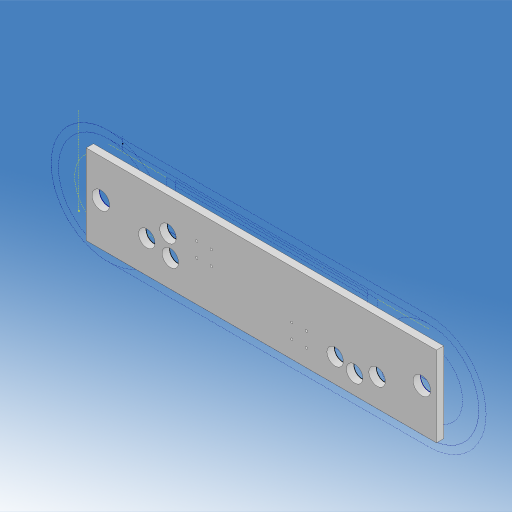
# Autodesk Inventor part: MasterSketch
Saved by Autodesk Inventor 2024 (Build 280153000, 153)
## iProperties
Created: 2024-03-21
Part Number: MasterSketch
Material: Generic
Document SubType Name: Modeling
Designer: seene
Density: 1 g/cm^3
Appearance: Default
Author: seene
Autodesk Inventor part; units mm, degrees
ref_plane "YZ Plane" through (0, 0, 0) normal (1, 0, 0) x (0, 1, 0)
ref_plane "XZ Plane" through (0, 0, 0) normal (0, 1, 0) x (-1, 0, 0)
ref_plane "XY Plane" through (0, 0, 0) normal (0, 0, 1) x (1, 0, 0)
sketch "Chassis" plane through (0, 0, 0) normal (0, 0, 1) x (1, 0, 0)
  line L0 (0, 0) -> (660.4, 0) construction
  line L1 (660.4, 0) -> (660.4, 152.4) construction
  line L2 (660.4, 152.4) -> (0, 152.4) construction
  line L3 (0, 152.4) -> (0, 0) construction
  line L4 (50.8, 127) -> (609.6, 127) construction
  line L5 (635, 101.6) -> (635, 50.8) construction
  line L6 (609.6, 25.4) -> (50.8, 25.4) construction
  line L7 (25.4, 50.8) -> (25.4, 101.6) construction
  arc A0 (50.8, 127) -> (25.4, 101.6) centre (50.8, 101.6) ccw construction
  arc A1 (25.4, 50.8) -> (50.8, 25.4) centre (50.8, 50.8) ccw construction
  arc A2 (609.6, 25.4) -> (635, 50.8) centre (609.6, 50.8) ccw construction
  arc A3 (635, 101.6) -> (609.6, 127) centre (609.6, 101.6) ccw construction
  dimension "d0" = 660.4
  dimension "d1" = 152.4
  dimension "d3" = 25.4
  dimension "d4" = 25.4
  constraints: 16 end point, 8 point on circle, 8 tangent, 4 centre point, 4 parallel, 3 equal radius, 2 perpendicular, 1 horizontal, 3 other
  measures "d0" distance of L2.end L1.end
  measures "d1" distance of L2.end L0.start
  measures "d3" distance between parallel lines of L2 L4
  measures "d4" radius of A0
sketch "Motor and motor mount" plane through (0, 0, 0) normal (0, 0, 1) x (1, 0, 0)
  line L0 (152.5322, 25.4) -> (519.6657, 25.4) construction
  line L1 (519.6657, 25.4) -> (519.6657, 127) construction
  line L2 (519.6657, 127) -> (152.5322, 127) construction
  line L3 (152.5322, 127) -> (152.5322, 25.4) construction
  line L4 (152.5322, 31.75) -> (519.6657, 31.75) construction
  line L5 (168.5983, 31.75) -> (502.5549, 31.75) construction
  line L6 (502.5549, 31.75) -> (502.5549, 131.1076) construction
  line L7 (502.5549, 131.1076) -> (168.5983, 131.1076) construction
  line L8 (168.5983, 131.1076) -> (168.5983, 31.75) construction
  circle A0 centre (459.6569, 62.4006) radius 45.974 construction
  line L9 (50.8, 127) -> (609.6, 127) construction
  line L10 (168.5983, 121.0746) -> (502.5549, 121.0746) construction
  line L11 (76.2661, 152.2106) -> (76.2661, 127) construction
  line L12 (0, 152.4) -> (0, 0) construction
  line L13 (609.6, 25.4) -> (50.8, 25.4) construction
  circle A1 centre (459.6569, 62.4006) radius 6.35 construction
  point P0 (76.2661, 139.6053)
  dimension "d77" = 13.97
  dimension "d5" = 367.1334
  dimension "d6" = 101.6
  dimension "d8" = 6.35
  dimension "d9" = 333.9566
  dimension "d10" = 17.1108
  dimension "d12" = 42.898
  dimension "d14" = 4.1076
  dimension "d15" = 5.9254
  dimension "d16" = 58.674
  dimension "d17" = 76.2661
  dimension "d18" = 76.2661
  dimension "d19" = 91.948
  dimension "d20" = 12.7
  constraints: 22 end point, 7 point on line, 4 horizontal, 4 parallel, 2 centre point, 2 perpendicular, 1 coincident, 1 midpoint, 1 vertical
  measures "d5" distance of L2.end L1.end
  measures "d6" distance of L1.end L0.end
  measures "d8" distance between parallel lines of L0 L4
  measures "d9" distance of L6.end L7.end
  measures "d10" distance between parallel lines of L1 L6
  measures "d12" distance from line of L6 A0.centre
  measures "d14" distance between parallel lines of L9 L7
  measures "d15" distance between parallel lines of L9 L10
  measures "d16" distance from line of A0.centre L10
  measures "d17" distance from line of point (76.266, 139.605) L12
  measures "d18" distance between parallel lines of L11 L3
  measures "d19" diameter of A0
  measures "d20" diameter of A1
sketch "Flipper drive rails" plane through (0, 0, 0) normal (0, 0, 1) x (1, 0, 0)
  circle A0 centre (609.6, 48.1766) radius 12.7 construction
  line L0 (660.4, 0) -> (660.4, 152.4) construction
  line L1 (0, 0) -> (660.4, 0) construction
  circle A1 centre (50.8, 48.1766) radius 12.7 construction
  line L2 (0, 152.4) -> (0, 0) construction
  circle A2 centre (50.8, 48.1766) radius 58.166 construction
  circle A3 centre (609.6, 48.1766) radius 58.166 construction
  circle A4 centre (459.6569, 62.4006) radius 45.974 construction
  dimension "d21" = 25.4
  dimension "d22" = 50.8
  dimension "d24" = 25.4
  dimension "d25" = 50.8
  dimension "d27" = 116.332
  dimension "d28" = 116.332
  dimension "d49" = 14.224
  constraints: 4 centre point, 2 coincident, 1 horizontal alignment
  measures "d21" diameter of A0
  measures "d22" distance from line of L0 A0.centre
  measures "d24" diameter of A1
  measures "d25" distance from line of A1.centre L2
  measures "d27" diameter of A2
  measures "d28" diameter of A3
  measures "d49" vertical distance of A0.centre A4.centre
sketch "Flipper Gears" plane through (0, 0, 0) normal (0, 0, 1) x (1, 0, 0)
  circle A0 centre (171.8512, 21.8146) radius 19.05 construction
  circle A1 centre (167.7675, 56.5) radius 15.875 construction
  circle A2 centre (130.9082, 30.7653) radius 22.86 construction
  circle A3 centre (130.9082, 30.7653) radius 23.8125 construction
  circle A4 centre (50.8, 48.1766) radius 58.166 construction
  circle A5 centre (609.6, 48.1766) radius 12.7 construction
  circle A6 centre (609.6, 48.1766) radius 86.36 construction
  circle A7 centre (531.7039, 22.629) radius 23.8125 construction
  circle A8 centre (531.7039, 22.629) radius 22.86 construction
  circle A9 centre (492.5049, 7.8006) radius 19.05 construction
  circle A10 centre (458.6619, 16.4266) radius 15.875 construction
  line L0 (203.8355, 81.25) -> (347.5395, 81.25) construction
  line L1 (347.5395, 81.25) -> (347.5395, 31.75) construction
  line L2 (347.5395, 31.75) -> (203.8355, 31.75) construction
  line L3 (203.8355, 31.75) -> (203.8355, 81.25) construction
  line L4 (422.5939, 16.4266) -> (458.6619, 16.4266) construction
  line L5 (167.7675, 56.5) -> (203.8355, 56.5) construction
  line L6 (278.8899, 41.1766) -> (422.5939, 41.1766) construction
  line L7 (422.5939, 41.1766) -> (422.5939, -8.3234) construction
  line L8 (422.5939, -8.3234) -> (278.8899, -8.3234) construction
  line L9 (278.8899, -8.3234) -> (278.8899, 41.1766) construction
  circle A11 centre (50.8, 48.1766) radius 86.36 construction
  line L10 (50.8, 48.1766) -> (609.6, 48.1766) construction
  line L11 (50.8, -50.8834) -> (609.6, -50.8834) construction
  line L12 (609.6, 147.2366) -> (50.8, 147.2366) construction
  arc A12 (50.8, 147.2366) -> (50.8, -50.8834) centre (50.8, 48.1766) ccw construction
  arc A13 (609.6, -50.8834) -> (609.6, 147.2366) centre (609.6, 48.1766) ccw construction
  circle A14 centre (50.8, 48.1766) radius 99.06 construction
  line L13 (50.8, 48.1766) -> (609.6, 48.1766) construction
  line L14 (50.8, -38.1834) -> (609.6, -38.1834) construction
  line L15 (609.6, 134.5366) -> (50.8, 134.5366) construction
  arc A15 (50.8, 134.5366) -> (50.8, -38.1834) centre (50.8, 48.1766) ccw construction
  arc A16 (609.6, -38.1834) -> (609.6, 134.5366) centre (609.6, 48.1766) ccw construction
  circle A17 centre (130.9082, 30.7653) radius 14.2875
  circle A18 centre (171.8512, 21.8146) radius 14.2875
  circle A19 centre (167.7675, 56.5) radius 14.2875
  circle A20 centre (458.6619, 16.4266) radius 14.224
  circle A21 centre (492.5049, 7.8006) radius 14.2875
  circle A22 centre (531.7039, 22.629) radius 14.2875
  circle A23 centre (50.8, 48.1766) radius 15.24
  circle A24 centre (609.6, 48.1766) radius 15.24
  circle A25 centre (217.8055, 70.1375) radius 2.0193
  circle A26 centre (243.2055, 70.1375) radius 2.0193
  circle A27 centre (217.8055, 44.7375) radius 2.0193
  circle A28 centre (243.2055, 44.7375) radius 2.0193
  circle A29 centre (408.6239, 30.0641) radius 2.0193
  circle A30 centre (408.6239, 4.6641) radius 2.0193
  circle A31 centre (383.2239, 30.0641) radius 2.0193
  circle A32 centre (383.2239, 4.6641) radius 2.0193
  circle A33 centre (609.6, 48.1766) radius 58.166 construction
  line L16 (168.5983, 31.75) -> (502.5549, 31.75) construction
  point P0 (0, 0)
  point P1 (330.2, 48.1766)
  point P2 (330.2, 48.1766)
  dimension "d29" = 38.1
  dimension "d30" = 31.75
  dimension "d31" = 45.72
  dimension "d32" = 47.625
  dimension "d34" = 172.72
  dimension "d35" = 47.625
  dimension "d36" = 45.72
  dimension "d37" = 38.1
  dimension "d38" = 31.75
  dimension "d39" = 143.704
  dimension "d43" = 36.068
  dimension "d50" = 31.75
  dimension "d52" = 143.704
  dimension "d54" = 36.068
  dimension "d60" = 172.72
  dimension "d62" = 12.7
  dimension "d63" = 28.575
  dimension "d64" = 28.575
  dimension "d65" = 28.575
  dimension "d66" = 28.448
  dimension "d67" = 28.575
  dimension "d68" = 28.575
  dimension "d69" = 30.48
  dimension "d70" = 30.48
  dimension "d76" = 4.0386
  dimension "d77" = 13.97
  dimension "d78" = 11.1125
  dimension "d81" = 25.4
  dimension "d84" = 25.4
  dimension "d87" = 4.0386
  dimension "d88" = 13.97
  dimension "d89" = 11.1125
  dimension "d92" = 25.4
  dimension "d95" = 25.4
  dimension "d98" = 116.332
  dimension "d99" = 49.5
  constraints: 36 end point, 32 centre point, 15 tangent, 13 coincident, 8 horizontal, 8 point on circle, 4 midpoint, 4 parallel, 3 perpendicular, 3 vertical, 1 collinear, 1 concentric, 12 other
  measures "d29" diameter of A0
  measures "d30" diameter of A1
  measures "d31" diameter of A2
  measures "d32" diameter of A3
  measures "d34" diameter of A6
  measures "d35" diameter of A7
  measures "d36" diameter of A8
  measures "d37" diameter of A9
  measures "d38" diameter of A10
  measures "d39" distance of L0.start L0.end
  measures "d43" distance from line of L3 L5.start
  measures "d50" vertical distance of A5.centre L4.end
  measures "d52" distance of L7.end L8.end
  measures "d54" distance from line of L4.end L7
  measures "d60" diameter of A11
  measures "d62" radial gap between concentric circles of A11 A14
  measures "d63" diameter of A17
  measures "d64" diameter of A18
  measures "d65" diameter of A19
  measures "d66" diameter of A20
  measures "d67" diameter of A21
  measures "d68" diameter of A22
  measures "d69" diameter of A23
  measures "d70" diameter of A24
  measures "d76" diameter of A25
  measures "d77" distance from line of A25.centre L3
  measures "d78" distance from line of L0 A25.centre
  measures "d81" distance of A25.centre A26.centre
  measures "d84" distance of A25.centre A27.centre
  measures "d87" diameter of A29
  measures "d88" distance from line of L7 A29.centre
  measures "d89" distance from line of L6 A29.centre
  measures "d92" distance of A29.centre A30.centre
  measures "d95" distance of A29.centre A31.centre
  measures "d98" diameter of A33
  measures "d99" distance between parallel lines of L2 L0
sketch "Flipper" plane through (0, 0, 0) normal (0, 0, 1) x (1, 0, 0)
  circle A0 centre (50.8, 48.1766) radius 63.5 construction
  circle A1 centre (-195.1482, 3.0916) radius 41.275 construction
  circle A2 centre (50.8, 48.1766) radius 86.36 construction
  line L0 (-195.1482, -38.1834) -> (50.8, -38.1834) construction
  point P0 (0, 0)
  point P1 (609.6, 48.1766)
  dimension "d57" = 82.55
  dimension "d58" = 172.72
  dimension "d56" = 127
  dimension "d59" = 245.9482
  constraints: 3 horizontal, 2 coincident, 2 end point, 2 vertical alignment, 1 centre point, 4 other
  measures "d56" diameter of A0
  measures "d59" horizontal distance of point (50.8, 48.177) point (-195.148, 3.092)
sketch "Sketch6" plane through (0, 0, 0) normal (0, 0, 1) x (1, 0, 0)
  line L0 (25.4, 114.3) -> (635, 114.3)
  line L1 (635, 114.3) -> (635, -25.4)
  line L2 (635, -25.4) -> (25.4, -25.4)
  line L3 (25.4, -25.4) -> (25.4, 114.3)
  circle A0 centre (609.6, 48.1766) radius 15.24 projected
  circle A1 centre (50.8, 48.1766) radius 15.24 projected
  circle A2 centre (130.9082, 30.7653) radius 14.2875 projected
  circle A3 centre (171.8512, 21.8146) radius 14.2875 projected
  circle A4 centre (167.7675, 56.5) radius 14.2875 projected
  circle A5 centre (458.6619, 16.4266) radius 14.224 projected
  circle A6 centre (492.5049, 7.8006) radius 14.2875 projected
  circle A7 centre (531.7039, 22.629) radius 14.2875 projected
  circle A8 centre (217.8055, 70.1375) radius 2.0193 projected
  circle A9 centre (217.8055, 44.7375) radius 2.0193 projected
  circle A10 centre (243.2055, 44.7375) radius 2.0193 projected
  circle A11 centre (243.2055, 70.1375) radius 2.0193 projected
  circle A12 centre (383.2239, 30.0641) radius 2.0193 projected
  circle A13 centre (408.6239, 30.0641) radius 2.0193 projected
  circle A14 centre (383.2239, 4.6641) radius 2.0193 projected
  circle A15 centre (408.6239, 4.6641) radius 2.0193 projected
  line L4 (50.8, 127) -> (609.6, 127) construction
  point P0 (0, 0)
  dimension "d72" = 139.7
  dimension "d73" = 25.4
  dimension "d101" = 12.7
  dimension "d104" = 25.4
  constraints: 4 end point, 2 horizontal, 1 parallel, 6 other
  measures "d72" distance between parallel lines of L2 L0
  measures "d101" distance between parallel lines of L0 L4
extrude "Extrusion1" add sketch "Sketch6" along normal blind 12.7
body "Solid1"
